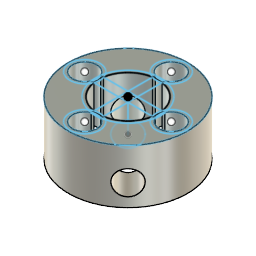
DIY7K_coupler (Autodesk Fusion 360 design; units mm, degrees)
Autodesk Fusion 360 part; units mm, degrees
sketch "スケッチ1" plane through (0, 0, 0) normal (0, 0, 1) x (1, 0, 0)
  circle A0 centre (0, 0) radius 11
  circle A1 centre (0, 8.0049) radius 2.25
  circle A2 centre (0, 8.0049) radius 2.75
  circle A3 centre (-8.0049, 0) radius 2.25
  circle A4 centre (-8.0049, 0) radius 2.75
  circle A5 centre (0, -8.0049) radius 2.25
  circle A6 centre (0, -8.0049) radius 2.75
  circle A7 centre (8.0049, 0) radius 2.25
  circle A8 centre (8.0049, 0) radius 2.75
  circle A9 centre (0, 0) radius 5.5
  circle A10 centre (0, 0) radius 6
  line L0 (-0.8817, 5.9349) -> (-0.8817, -5.9349)
  line L1 (-0.8817, -5.9349) -> (0.8817, -5.9349)
  line L2 (0.8817, -5.9349) -> (0.8817, 5.9349)
  line L3 (-5.9349, 0.8817) -> (5.9349, 0.8817)
  line L4 (5.9349, 0.8817) -> (5.9349, -0.8817)
  line L5 (5.9349, -0.8817) -> (-5.9349, -0.8817)
  dimension "d1" = 4.5
  dimension "d2" = 5.5
  dimension "d4" = 360
  dimension "d10" = 11
  constraint coincident A0.centre A9.centre
  constraint concentric A1 A2
  constraint concentric A0 A10
  constraint coincident A1 L0.start
  constraint coincident A10 L0.start
  constraint coincident A5 L0.end
  constraint coincident A10 L0.end
  constraint vertical L0
  constraint coincident A5 L1.end
  constraint coincident A10 L1.end
  constraint coincident A10 L2.end
  constraint coincident A1 L2.end
  constraint coincident A3 L3.start
  constraint coincident A10 L3.start
  constraint coincident A7 L3.end
  constraint coincident A10 L3.end
  constraint coincident A7 L4.end
  constraint coincident A10 L4.end
  constraint coincident A10 L5.end
  constraint coincident A3 L5.end
  measures "d1" diameter of A1
  measures "d2" diameter of A2
  measures "d10" diameter of A9
extrude "押し出し1" add sketch "スケッチ1" against normal blind 10 contours A0 | A1 A2 A10 | A2 A9 A10 L0 | A1 A9 L0 L2 | A2 A9 A10 L2 | A2 A4 A9 A10 | A2 A9 L0 | A2 A9 L0 L2 | A2 A8 A9 A10 | A2 A9 L2 | A2 A4 A9 L0 L3 | A3 A4 A10 | A4 A9 A10 L3 | A2 L0 L2 L3 | A2 A8 A9 L2 L3 | A8 A9 A10 L3 | A7 A8 A10 | A4 A9 L3 | A4 A9 A10 L5 | A4 A6 A9 A10 | A3 A9 L3 L5 | L0 L2 L3 L5 | A4 L0 L3 L5 | A8 A9 L3 | A7 A9 L3 L5 | A8 L2 L3 L5 | A4 A9 L3 L5 | A4 A9 L5 | A4 A6 A9 L0 L5 | A5 A6 A10 | A6 A9 A10 L0 | A6 L0 L2 L5 | A8 A9 L3 L5 | A6 A8 A9 A10 | A8 A9 A10 L5 | A6 A8 A9 L2 L5 | A6 A9 L0 | A5 A9 L0 L2 | A6 A9 L0 L2 | A8 A9 L5 | A6 A9 A10 L2 | A6 A9 L2
sketch "スケッチ2" plane through (0, 0, 0) normal (1, 0, 0) x (0, 1, 0)
  line L0 (0, 0) -> (0, -6)
  circle A0 through (1.591, -6, 1.591) (-0.7955, -4.0514, -0.7955) (-0.7955, -7.9486, -0.7955)
  dimension "d7" = 4.5
  constraint coincident L0.start origin
extrude "押し出し2" cut sketch "スケッチ2" against normal mid plane 32 contours A0 in plane through (0, 0, 0) normal (-0.707107, 0.707107, 0)
extrude "押し出し3" cut sketch "スケッチ1" against normal blind 10 contours A2 A9 L0 | A2 A9 L0 L2 | A2 A9 L2 | A2 A4 A9 L0 L3 | A2 L0 L2 L3 | A2 A8 A9 L2 L3 | A4 A9 L3 | L0 L2 L3 L5 | A4 L0 L3 L5 | A8 A9 L3 | A8 L2 L3 L5 | A4 A9 L3 L5 | A4 A9 L5 | A4 A6 A9 L0 L5 | A6 L0 L2 L5 | A8 A9 L3 L5 | A6 A8 A9 L2 L5 | A6 A9 L0 | A6 A9 L0 L2 | A8 A9 L5 | A6 A9 L2
extrude "押し出し4" cut sketch "スケッチ1" against normal blind 14 contours A1 A9 L0 L2 | A3 A9 L3 L5 | A7 A9 L3 L5 | A5 A9 L0 L2
